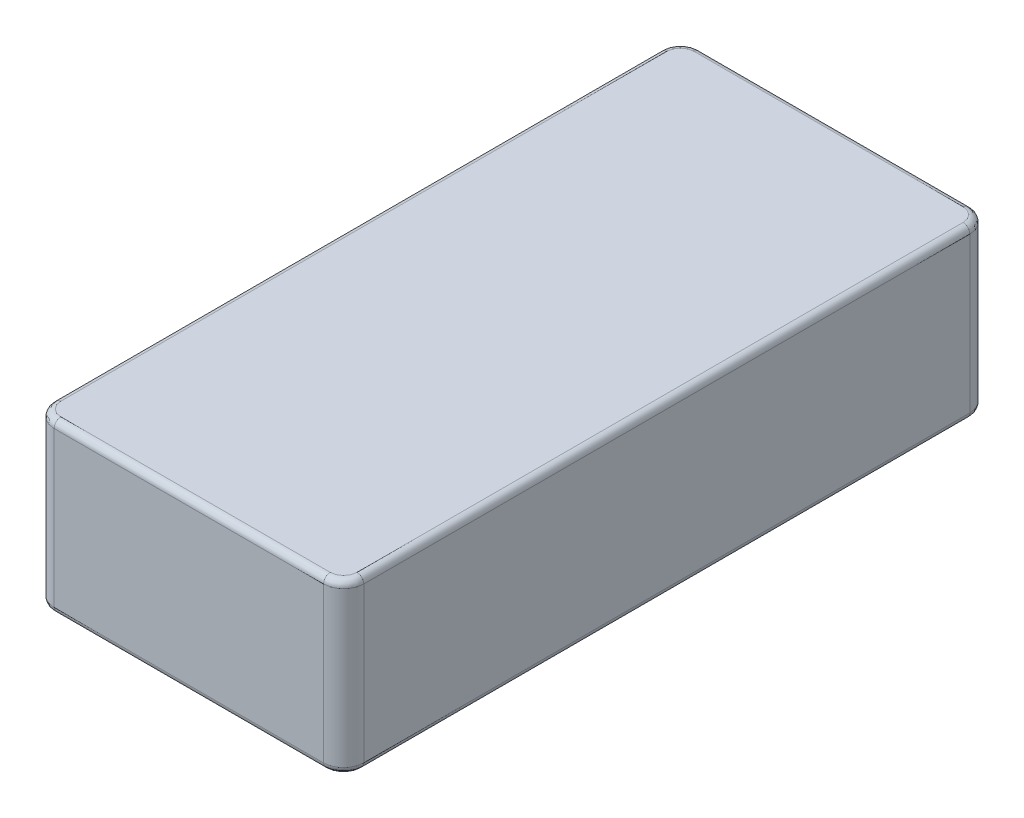
# Autodesk Inventor part: battery
Saved by Autodesk Inventor 2022.2 (Build 262287000, 287)
## iProperties
Created: 2021-01-30
Part Number: battery
Material: Generic
Document SubType Name: Modeling
Designer: User
Density: 1 g/cm^3
Appearance: Default
Author: User
Autodesk Inventor part; units mm, degrees
ref_plane "YZ Plane" through (0, 0, 0) normal (1, 0, 0) x (0, 1, 0)
ref_plane "XZ Plane" through (0, 0, 0) normal (0, 1, 0) x (-1, 0, 0)
ref_plane "XY Plane" through (0, 0, 0) normal (0, 0, 1) x (1, 0, 0)
sketch "Sketch1" plane through (0, 0, 0) normal (0, 1, 0) x (-1, 0, 0)
  line L0 (20, 48) -> (-20, 48)
  line L1 (-23, 45) -> (-23, -45)
  line L2 (-20, -48) -> (20, -48)
  line L3 (23, -45) -> (23, 45)
  line L4 (23, 48) -> (-23, -48) construction
  line L5 (-23, 48) -> (23, -48) construction
  arc A0 (23, 45) -> (20, 48) centre (20, 45) ccw
  arc A1 (20, -48) -> (23, -45) centre (20, -45) ccw
  arc A2 (-23, -45) -> (-20, -48) centre (-20, -45) ccw
  arc A3 (-20, 48) -> (-23, 45) centre (-20, 45) ccw
  circle A4 centre (-16, 43.5) radius 2
  line L6 (0, 48) -> (0, 45)
  circle A5 centre (16, 43.5) radius 2
  point P0 (0, 0)
  dimension "d0" = 46
  dimension "d1" = 96
  dimension "d2" = 3
  dimension "d7" = 4
  dimension "d8" = 7
  dimension "d9" = 4.5
  constraints: 14 end point, 8 point on circle, 8 point on line, 8 tangent, 6 centre point, 3 equal radius, 3 midpoint, 2 parallel, 1 horizontal, 1 perpendicular, 1 symmetric about line, 1 vertical, 1 other
  measures "d0" distance of L5.end L4.end
  measures "d1" distance of L4.end L5.start
  measures "d2" radius of A0
  measures "d7" diameter of A4
  measures "d8" distance from line of L1 A4.centre
  measures "d9" distance from line of L0 A4.centre
extrude "Extrusion1" add sketch "Sketch1" along normal blind 25 contours A0 L3 A1 L2 A2 L1 A3 L0 | A4 | A5
fillet "Fillet1" radius 1 16 edges at (22.1213, 25, -47.1213) (0, 25, -48) (-22.1213, 25, -47.1213) (-23, 25, 0) (-22.1213, 25, 47.1213) (0, 25, 48) (22.1213, 25, 47.1213) (23, 25, 0) (22.1213, 0, -47.1213) (0, 0, -48) (-22.1213, 0, -47.1213) (-23, 0, 0) (-22.1213, 0, 47.1213) (0, 0, 48) (22.1213, 0, 47.1213) (23, 0, 0)
extrude "Extrusion2" cut sketch "Sketch1" along normal blind 20 contours A4 | A5
sketch "Sketch2" plane through (0, 25, 0) normal (0, 1, 0) x (1, 0, 0)
  line L0 (21, 40) -> (21, -42.2706) construction
  line L1 (21, -42.2706) -> (-20.9862, -42.2706) construction
  line L2 (-20.9862, -42.2706) -> (-20.9862, 40) construction
  line L3 (-20.9862, 40) -> (21, 40) construction
  point P0 (0, 0)
  constraints: 2 other
body "Solid1"
